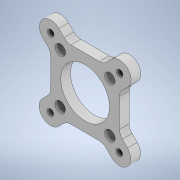
# Autodesk Inventor part: encoder_shelf_1
Saved by Autodesk Inventor 2020 (Build 240168000, 168)
## iProperties
Created: 2020-10-12
Part Number: encoder_shelf_1
Material: Generic
Document SubType Name: Modeling
Designer: Shuang Peng
Density: 1 g/cm^3
Appearance: Default
Author: Shuang Peng
Autodesk Inventor part; units mm, degrees
ref_plane "YZ Plane" through (0, 0, 0) normal (1, 0, 0) x (0, 1, 0)
ref_plane "XZ Plane" through (0, 0, 0) normal (0, 1, 0) x (-1, 0, 0)
ref_plane "XY Plane" through (0, 0, 0) normal (0, 0, 1) x (1, 0, 0)
sketch "Sketch1" plane through (0, 0, 0) normal (0, 0, 1) x (1, 0, 0)
  circle A0 centre (1.7602, -3.9548) radius 0.175 projected
  circle A1 centre (1.9888, 2.9032) radius 0.175 projected
  circle A2 centre (4.9606, -1.2116) radius 0.175 projected
  circle A3 centre (0.16, -0.7544) radius 0.175 projected
  circle A4 centre (-7.1552, -3.4976) radius 0.175 projected
  circle A5 centre (-6.2408, 1.303) radius 0.175 projected
  circle A6 centre (7.653, -7.587) radius 1.0033 projected
  circle A7 centre (-7.587, -7.587) radius 1.0033 projected
  circle A8 centre (-7.587, 7.653) radius 1.0033 projected
  circle A9 centre (7.653, 7.653) radius 1.0033 projected
  circle A10 centre (-7.1552, 1.9888) radius 0.175 projected
  circle A11 centre (-7.3838, -1.6688) radius 0.175 projected
  circle A12 centre (-3.9548, -1.4402) radius 0.175 projected
  circle A13 centre (5.6464, -0.5258) radius 0.175 projected
  circle A14 centre (6.5608, 0.3886) radius 0.175 projected
  circle A15 centre (-0.7544, -1.2116) radius 0.175 projected
  circle A16 centre (4.2748, 0.16) radius 0.175 projected
  line L0 (-10, 10) -> (-10, -10) projected
  line L1 (-10, -10) -> (10, -10) projected
  line L2 (10, -10) -> (10, 10) projected
  line L3 (10, 10) -> (-10, 10) projected
  circle A17 centre (-7.587, 7.653) radius 1.5
  circle A18 centre (7.653, 7.653) radius 1.5
  circle A19 centre (-7.587, -7.587) radius 1.5
  circle A20 centre (7.653, -7.587) radius 1.5
  line L4 (0, 0) -> (-7.587, 7.653)
  line L5 (0, 0) -> (-10.5606, 10.6524)
  circle A21 centre (-10.5606, 10.6524) radius 2.5
  circle A22 centre (-10.5606, 10.6524) radius 1
  circle A23 centre (0, 0) radius 7.5
  circle A24 centre (-10.6524, -10.5606) radius 2.5
  circle A25 centre (-10.6524, -10.5606) radius 1
  line L6 (0, 0) -> (-10.6524, -10.5606)
  circle A26 centre (-7.653, -7.587) radius 1.5
  circle A27 centre (10.5606, -10.6524) radius 2.5
  circle A28 centre (10.5606, -10.6524) radius 1
  line L7 (0, 0) -> (10.5606, -10.6524)
  circle A29 centre (7.587, -7.653) radius 1.5
  circle A30 centre (10.6524, 10.5606) radius 2.5
  circle A31 centre (10.6524, 10.5606) radius 1
  line L8 (0, 0) -> (10.6524, 10.5606)
  circle A32 centre (7.653, 7.587) radius 1.5
  line L9 (0, 0) -> (-10.5606, 10.6524) construction
  line L10 (2.4856, 2.4641) -> (-8.075, 13.1166)
  line L11 (-13.0461, 8.1883) -> (-2.4856, -2.4641)
  arc A33 (-2.4856, -2.4641) -> (2.4856, 2.4641) centre (0, 0) ccw
  arc A34 (-8.075, 13.1166) -> (-13.0461, 8.1883) centre (-10.5606, 10.6524) ccw
  line L12 (0, 0) -> (10.6524, 10.5606) construction
  line L13 (2.4641, -2.4856) -> (13.1166, 8.075)
  line L14 (8.1883, 13.0461) -> (-2.4641, 2.4856)
  arc A35 (-2.4641, 2.4856) -> (2.4641, -2.4856) centre (0, 0) ccw
  arc A36 (13.1166, 8.075) -> (8.1883, 13.0461) centre (10.6524, 10.5606) ccw
  line L15 (0, 0) -> (10.5606, -10.6524) construction
  line L16 (-2.4856, -2.4641) -> (8.075, -13.1166)
  line L17 (13.0461, -8.1883) -> (2.4856, 2.4641)
  arc A37 (2.4856, 2.4641) -> (-2.4856, -2.4641) centre (0, 0) ccw
  arc A38 (8.075, -13.1166) -> (13.0461, -8.1883) centre (10.5606, -10.6524) ccw
  line L18 (0, 0) -> (-10.6524, -10.5606) construction
  line L19 (-2.4641, 2.4856) -> (-13.1166, -8.075)
  line L20 (-8.1883, -13.0461) -> (2.4641, -2.4856)
  arc A39 (2.4641, -2.4856) -> (-2.4641, 2.4856) centre (0, 0) ccw
  arc A40 (-13.1166, -8.075) -> (-8.1883, -13.0461) centre (-10.6524, -10.5606) ccw
  circle A41 centre (0, 0) radius 12
  point P0 (-5.2803, 5.3262)
  point P1 (5.3262, 5.2803)
  point P2 (5.2803, -5.3262)
  point P3 (-5.3262, -5.2803)
  point P4 (9.1526, 7.62)
  point P5 (6.1534, 7.62)
  point P6 (-7.62, -9.0866)
  point P7 (-7.62, -6.0874)
  point P8 (10.5667, -5.6873)
  point P9 (10.6155, 5.5955)
  point P10 (5.6873, 10.5667)
  point P11 (-5.5955, 10.6155)
  point P12 (-10.5667, 5.6873)
  point P13 (-10.6155, -5.5955)
  point P14 (-5.6873, -10.5667)
  point P15 (5.5955, -10.6155)
  point P16 (6.5599, -6.5599)
  point P17 (8.6801, -8.6801)
  point P18 (-7.2786, -1.8087)
  point P19 (-7.349, -1.4973)
  point P20 (-7.2672, 1.8543)
  point P21 (-7.1817, 2.1618)
  dimension "d0" = 3
  dimension "d1" = 3
  dimension "d2" = 3
  dimension "d3" = 3
  dimension "d5" = 15
  dimension "d6" = 5
  dimension "d7" = 2
  dimension "d8" = 15
  dimension "d11" = 360
  dimension "d13" = 7
  dimension "d14" = 7
  dimension "d15" = 7
  dimension "d16" = 7
  dimension "d17" = 24
  constraints: 42 end point, 25 centre point, 16 coincident, 16 point on circle, 16 tangent, 4 collinear, 4 midpoint, 4 parallel, 1 perpendicular, 35 other
  measures "d0" diameter of A17
  measures "d1" diameter of A18
  measures "d2" diameter of A19
  measures "d3" diameter of A20
  measures "d5" distance of L4.start L5.end
  measures "d6" diameter of A21
  measures "d7" diameter of A22
  measures "d8" diameter of A23
  measures "d13" diameter of A34
  measures "d14" diameter of A36
  measures "d15" diameter of A38
  measures "d16" diameter of A40
  measures "d17" diameter of A41
extrude "Extrusion1" add sketch "Sketch1" along normal blind 3 contours L10 L3 L14 A23 | A23 L4 A17 A41 L3 L10 | L14 L3 A41 A18 A32 L8 A23 | L8 A32 A18 A41 L2 L13 A23 | A23 L11 L0 A41 A17 L4 | L10 A41 L14 L3 | L3 A41 L10 | L14 A41 L3 | L13 L2 L17 A23 | L7 A29 A41 L1 L16 A23 | A23 L17 L2 A41 A20 L7 | A23 A10 A11 L19 L0 L11 | L6 A19 A26 A41 L0 L19 A23 | A23 L20 L1 A41 A26 A19 L6 | A41 A17 L5 A21 L3 | L3 A21 L0 A41 L11 A34 L10 | A41 L14 A36 L13 L2 A30 L3 | L3 A30 L8 A18 A41 | L13 A41 L17 L2 | L2 A41 L13 | L16 L1 L20 A23 | A41 L0 A21 L5 A17 | L11 A41 L0 | L0 L19 A41 L11 | L0 A41 L19 | A21 L5 A22 L3 | L3 A22 L0 A21 | A30 L2 A31 L3 | L3 A31 L8 A30 | L17 A41 L2 | A41 A18 L8 A30 L2 | L16 A41 L20 L1 | L1 A41 L16 | A29 L7 A27 L1 A41 | L20 A41 L1 | A41 A26 L6 A24 L0 | L0 A24 L1 A41 L20 A40 L19 | A21 L0 A22 L5 | L8 A31 L2 A30 | A41 L17 A38 L16 L1 A27 L2 | L2 A27 L7 A20 A41 | L1 A24 L6 A26 A41 | A24 L6 A25 L0 | L0 A25 L1 A24 | A27 L1 A28 L2 | L2 A28 L7 A27 | A27 L7 A28 L1 | L1 A25 L6 A24
sketch "Sketch2" plane through (0, 0, 3) normal (0, 0, 1) x (1, 0, 0)
  arc A0 (13.1166, 8.075) -> (8.1883, 13.0461) centre (10.6524, 10.5606) ccw projected
  line L0 (8.1883, 13.0461) -> (5.6873, 10.5667) projected
  arc A1 (5.6873, 10.5667) -> (-5.5955, 10.6155) centre (0, 0) ccw projected
  line L1 (-5.5955, 10.6155) -> (-8.075, 13.1166) projected
  arc A2 (-8.075, 13.1166) -> (-13.0461, 8.1883) centre (-10.5606, 10.6524) ccw projected
  line L2 (-13.0461, 8.1883) -> (-10.5667, 5.6873) projected
  arc A3 (-10.5667, 5.6873) -> (-10.6155, -5.5955) centre (0, 0) ccw projected
  line L3 (-10.6155, -5.5955) -> (-13.1166, -8.075) projected
  arc A4 (-13.1166, -8.075) -> (-8.1883, -13.0461) centre (-10.6524, -10.5606) ccw projected
  line L4 (-8.1883, -13.0461) -> (-5.6873, -10.5667) projected
  arc A5 (-5.6873, -10.5667) -> (5.5955, -10.6155) centre (0, 0) ccw projected
  line L5 (5.5955, -10.6155) -> (8.075, -13.1166) projected
  arc A6 (8.075, -13.1166) -> (13.0461, -8.1883) centre (10.5606, -10.6524) ccw projected
  line L6 (13.0461, -8.1883) -> (10.5667, -5.6873) projected
  arc A7 (10.5667, -5.6873) -> (10.6155, 5.5955) centre (0, 0) ccw projected
  line L7 (10.6155, 5.5955) -> (13.1166, 8.075) projected
  circle A8 centre (-10.6524, -10.5606) radius 1 projected
  circle A9 centre (-7.587, 7.653) radius 1.5 projected
  arc A10 (9.1526, 7.62) -> (6.1534, 7.62) centre (7.653, 7.653) ccw projected
  arc A11 (6.1534, 7.62) -> (9.1526, 7.62) centre (7.653, 7.587) ccw projected
  arc A12 (-7.62, -6.0874) -> (-7.62, -9.0866) centre (-7.653, -7.587) ccw projected
  arc A13 (-7.62, -9.0866) -> (-7.62, -6.0874) centre (-7.587, -7.587) ccw projected
  circle A14 centre (-7.1552, -3.4976) radius 0.175 projected
  circle A15 centre (10.5606, -10.6524) radius 1 projected
  arc A16 (8.6801, -8.6801) -> (6.5599, -6.5599) centre (7.653, -7.587) ccw projected
  arc A17 (6.5599, -6.5599) -> (8.6801, -8.6801) centre (7.587, -7.653) ccw projected
  arc A18 (-7.2786, -1.8087) -> (-7.1817, 2.1618) centre (0, 0) ccw projected
  arc A19 (-7.349, -1.4973) -> (-7.2786, -1.8087) centre (-7.3838, -1.6688) ccw projected
  arc A20 (-7.2672, 1.8543) -> (-7.349, -1.4973) centre (0, 0) ccw projected
  arc A21 (-7.1817, 2.1618) -> (-7.2672, 1.8543) centre (-7.1552, 1.9888) ccw projected
  circle A22 centre (10.6524, 10.5606) radius 1 projected
  circle A23 centre (-10.5606, 10.6524) radius 1 projected
  circle A24 centre (0, 0) radius 7.5
  point P0 (-7.2672, 1.8543)
  point P1 (-7.1817, 2.1618)
  point P2 (-7.2786, -1.8087)
  dimension "d20" = 15
  constraints: 1 centre point, 1 coincident
  measures "d20" diameter of A24
extrude "Extrusion2" add sketch "Sketch2" against normal blind 3 contours A14 | A19 A24 | A24 A21
sketch "Sketch3" plane through (0, 0, 3) normal (0, 0, 1) x (1, 0, 0)
  arc A0 (13.1166, 8.075) -> (8.1883, 13.0461) centre (10.6524, 10.5606) ccw projected
  line L0 (8.1883, 13.0461) -> (5.6873, 10.5667) projected
  arc A1 (5.6873, 10.5667) -> (-5.5955, 10.6155) centre (0, 0) ccw projected
  line L1 (-5.5955, 10.6155) -> (-8.075, 13.1166) projected
  arc A2 (-8.075, 13.1166) -> (-13.0461, 8.1883) centre (-10.5606, 10.6524) ccw projected
  line L2 (-13.0461, 8.1883) -> (-10.5667, 5.6873) projected
  arc A3 (-10.5667, 5.6873) -> (-10.6155, -5.5955) centre (0, 0) ccw projected
  line L3 (-10.6155, -5.5955) -> (-13.1166, -8.075) projected
  arc A4 (-13.1166, -8.075) -> (-8.1883, -13.0461) centre (-10.6524, -10.5606) ccw projected
  line L4 (-8.1883, -13.0461) -> (-5.6873, -10.5667) projected
  arc A5 (-5.6873, -10.5667) -> (5.5955, -10.6155) centre (0, 0) ccw projected
  line L5 (5.5955, -10.6155) -> (8.075, -13.1166) projected
  arc A6 (8.075, -13.1166) -> (13.0461, -8.1883) centre (10.5606, -10.6524) ccw projected
  line L6 (13.0461, -8.1883) -> (10.5667, -5.6873) projected
  arc A7 (10.5667, -5.6873) -> (10.6155, 5.5955) centre (0, 0) ccw projected
  line L7 (10.6155, 5.5955) -> (13.1166, 8.075) projected
  circle A8 centre (-10.6524, -10.5606) radius 1 projected
  circle A9 centre (-7.587, 7.653) radius 1.5 projected
  arc A10 (9.1526, 7.62) -> (6.1534, 7.62) centre (7.653, 7.653) ccw projected
  arc A11 (6.1534, 7.62) -> (9.1526, 7.62) centre (7.653, 7.587) ccw projected
  arc A12 (-7.62, -6.0874) -> (-7.62, -9.0866) centre (-7.653, -7.587) ccw projected
  arc A13 (-7.62, -9.0866) -> (-7.62, -6.0874) centre (-7.587, -7.587) ccw projected
  circle A14 centre (10.5606, -10.6524) radius 1 projected
  arc A15 (8.6801, -8.6801) -> (6.5599, -6.5599) centre (7.653, -7.587) ccw projected
  arc A16 (6.5599, -6.5599) -> (8.6801, -8.6801) centre (7.587, -7.653) ccw projected
  circle A17 centre (0, 0) radius 7.5 projected
  circle A18 centre (10.6524, 10.5606) radius 1 projected
  circle A19 centre (-10.5606, 10.6524) radius 1 projected
  line L8 (-5.5955, 10.6155) -> (-8.075, 13.1166) projected
  line L9 (8.1883, 13.0461) -> (5.6873, 10.5667) projected
  line L10 (-5.5955, 10.6155) -> (5.6873, 10.5667)
  arc A20 (-10.5667, 5.6873) -> (-10.6155, -5.5955) centre (0, 0) ccw projected
  line L11 (-10.5667, 5.6873) -> (-10.6155, -5.5955)
  line L12 (-5.6873, -10.5667) -> (5.5955, -10.6155)
  line L13 (10.5667, -5.6873) -> (10.6155, 5.5955)
  constraints: 8 end point
extrude "Extrusion3" cut sketch "Sketch3" against normal blind 3 contours A7 L13 | L10 A1 | A5 L12 | L11 A3
fillet "Fillet2" radius 3 8 edges at (-10.5667, 5.6873, 1.5) (-10.6155, -5.5955, 1.5) (-5.6873, -10.5667, 1.5) (5.5955, -10.6155, 1.5) (10.5667, -5.6873, 1.5) (10.6155, 5.5955, 1.5) (5.6873, 10.5667, 1.5) (-5.5955, 10.6155, 1.5)
sketch "Sketch4" plane through (0, 0, 3) normal (0, 0, 1) x (1, 0, 0)
  line L0 (-4.4447, -10.5721) -> (4.3529, -10.6102) projected
  arc A0 (6.4704, -11.498) -> (4.3529, -10.6102) centre (4.3399, -13.6101) ccw projected
  line L1 (6.4704, -11.498) -> (8.075, -13.1166) projected
  arc A1 (8.075, -13.1166) -> (13.0461, -8.1883) centre (10.5606, -10.6524) ccw projected
  line L2 (13.0461, -8.1883) -> (11.4416, -6.5698) projected
  arc A2 (10.5721, -4.4447) -> (11.4416, -6.5698) centre (13.572, -4.4576) ccw projected
  line L3 (10.5721, -4.4447) -> (10.6102, 4.3529) projected
  arc A3 (11.498, 6.4704) -> (10.6102, 4.3529) centre (13.6101, 4.3399) ccw projected
  line L4 (11.498, 6.4704) -> (13.1166, 8.075) projected
  arc A4 (13.1166, 8.075) -> (8.1883, 13.0461) centre (10.6524, 10.5606) ccw projected
  line L5 (8.1883, 13.0461) -> (6.5698, 11.4416) projected
  arc A5 (4.4447, 10.5721) -> (6.5698, 11.4416) centre (4.4576, 13.572) ccw projected
  line L6 (4.4447, 10.5721) -> (-4.3529, 10.6102) projected
  arc A6 (-6.4704, 11.498) -> (-4.3529, 10.6102) centre (-4.3399, 13.6101) ccw projected
  line L7 (-6.4704, 11.498) -> (-8.075, 13.1166) projected
  arc A7 (-8.075, 13.1166) -> (-13.0461, 8.1883) centre (-10.5606, 10.6524) ccw projected
  line L8 (-13.0461, 8.1883) -> (-11.4416, 6.5698) projected
  arc A8 (-10.5721, 4.4447) -> (-11.4416, 6.5698) centre (-13.572, 4.4576) ccw projected
  line L9 (-10.5721, 4.4447) -> (-10.6102, -4.3529) projected
  arc A9 (-11.498, -6.4704) -> (-10.6102, -4.3529) centre (-13.6101, -4.3399) ccw projected
  line L10 (-11.498, -6.4704) -> (-13.1166, -8.075) projected
  arc A10 (-13.1166, -8.075) -> (-8.1883, -13.0461) centre (-10.6524, -10.5606) ccw projected
  line L11 (-8.1883, -13.0461) -> (-6.5698, -11.4416) projected
  arc A11 (-4.4447, -10.5721) -> (-6.5698, -11.4416) centre (-4.4576, -13.572) ccw projected
  circle A12 centre (-10.6524, -10.5606) radius 1 projected
  circle A13 centre (-7.587, 7.653) radius 1.5 projected
  arc A14 (9.1526, 7.62) -> (6.1534, 7.62) centre (7.653, 7.653) ccw projected
  arc A15 (6.1534, 7.62) -> (9.1526, 7.62) centre (7.653, 7.587) ccw projected
  arc A16 (-7.62, -6.0874) -> (-7.62, -9.0866) centre (-7.653, -7.587) ccw projected
  arc A17 (-7.62, -9.0866) -> (-7.62, -6.0874) centre (-7.587, -7.587) ccw projected
  circle A18 centre (10.5606, -10.6524) radius 1 projected
  arc A19 (8.6801, -8.6801) -> (6.5599, -6.5599) centre (7.653, -7.587) ccw projected
  arc A20 (6.5599, -6.5599) -> (8.6801, -8.6801) centre (7.587, -7.653) ccw projected
  circle A21 centre (0, 0) radius 7.5 projected
  circle A22 centre (10.6524, 10.5606) radius 1 projected
  circle A23 centre (-10.5606, 10.6524) radius 1 projected
  circle A24 centre (-7.653, -7.587) radius 1.6
  circle A25 centre (-7.587, 7.653) radius 1.6
  circle A26 centre (7.653, -7.587) radius 1.6
  circle A27 centre (7.653, 7.653) radius 1.6
  dimension "d27" = 3.2
  dimension "d28" = 3.2
  dimension "d29" = 3.2
  dimension "d30" = 3.2
  constraints: 4 centre point, 4 coincident
  measures "d27" diameter of A24
  measures "d28" diameter of A25
  measures "d29" diameter of A26
  measures "d30" diameter of A27
extrude "Extrusion4" cut sketch "Sketch4" against normal blind 3 contours A24 | A25 | A26 | A27
body "Solid1"
